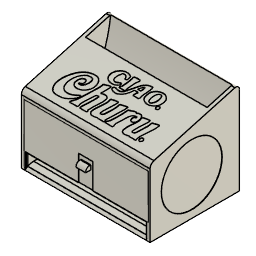
assembled chiky (Autodesk Fusion 360 design; units mm, degrees)
part number: 2026-06-02-16-31-48-869
part number: 2026-06-07-23-37-08-054
Autodesk Fusion 360 part; units mm, degrees
note: some values were not read from the file. Chosen so that the rebuilt part matches the saved one: that a step has no effect.
(part 1 of 7)
sketch "Sketch1" plane through (0, 0, 0) normal (0, 0, 1) x (1, 0, 0)
  line L0 (-170, 30) -> (0, 30)
  line L1 (0, 30) -> (0, 0)
  line L2 (0, 0) -> (-170, 0)
  line L3 (-170, 0) -> (-170, 30)
  spline S0 degree 3 poles (7.5215, 61.624) (7.5215, 61.5088) (7.5215, 61.3936) (7.5215, 61.2749) knots 0 0 0 0 1 1 1 1
  constraint horizontal L0
  constraint vertical L1
  constraint horizontal L2
  constraint vertical L3
  constraint coincident L1.end L2.start
sketch "Sketch2" plane through (0, 0, 15) normal (0, 0, 1) x (-1, 0, 0)
  line L0 (170, 0) -> (0, 0)
  line L1 (0, 0) -> (0, -30)
  line L2 (0, -30) -> (170, -30)
  line L3 (170, -30) -> (170, 0)
  line L4 (0, 0) -> (170, 0)
  line L5 (170, 0) -> (170, 30)
  line L6 (170, 30) -> (0, 30)
  line L7 (0, 30) -> (0, 0)
  constraint horizontal L4
  constraint vertical L5
  constraint horizontal L6
  constraint vertical L7
  constraint coincident L0.end L1.start
sketch "Sketch3" plane through (0, 0, 15) normal (0, 0, 1) x (-1, 0, 0)
sketch "Sketch4" plane through (0, 0, 0) normal (1, 0, 0) x (0, 1, 0)
sketch "Sketch5" plane through (0, 0, 0) normal (1, 0, 0) x (0, 1, 0)
  line L0 (0, 0) -> (-70, 0)
  line L1 (-70, 0) -> (-70, 150)
  line L2 (-70, 150) -> (0, 150)
  line L3 (0, 150) -> (0, 0)
  constraint horizontal L0
  constraint vertical L1
  constraint horizontal L2
  constraint vertical L3
  constraint coincident L0.start L3.end
sketch "Sketch6" plane through (0, 0, 0) normal (1, 0, 0) x (0, 1, 0)
sketch "Sketch7" plane through (0, 0, 0) normal (1, 0, 0) x (0, 1, 0)
sketch "Sketch8" plane through (-170, 0, 0) normal (-1, 0, 0) x (0, -1, 0)
  line L0 (0, 0) -> (70, 0)
  line L1 (70, 0) -> (70, 150)
  line L2 (70, 150) -> (0, 150)
  line L3 (0, 150) -> (0, 0)
  line L4 (0, 0) -> (70, 150)
  line L5 (0, 150) -> (0, 0)
  constraint coincident L0.start L3.end
  constraint coincident L1.end L2.start
  constraint coincident L2.end L3.start
sketch "Sketch9" plane through (0, 0, 0) normal (0, 1, 0) x (1, 0, 0)
sketch "Sketch10" plane through (0, 0, 0) normal (0, 1, 0) x (1, 0, 0)
sketch "Sketch11" plane through (0, 0, 0) normal (0, 0, 1) x (1, 0, 0)
  line L0 (100, -50) -> (-80, -50)
  line L1 (-80, -50) -> (-80, 0)
  line L2 (-80, 0) -> (100, 0)
  line L3 (100, 0) -> (100, -50)
  constraint horizontal L0
  constraint vertical L1
  constraint horizontal L2
  constraint vertical L3
sketch "Sketch12" plane through (0, 0, 0) normal (0, 0, 1) x (1, 0, 0)
  line L0 (170.2577, -0.0482) -> (0.2577, -0.0482)
  line L1 (0.2577, -0.0482) -> (0.2577, 119.9518)
  line L2 (0.2577, 119.9518) -> (170.2577, 119.9518)
  line L3 (170.2577, 119.9518) -> (170.2577, -0.0482)
  dimension "d12" = 170
  dimension "d13" = 120
  constraint horizontal L0
  constraint vertical L1
  constraint horizontal L2
  constraint vertical L3
  measures "d12" distance of L0.start L0.end
  measures "d13" distance of L0.start L2.end
sketch "Sketch13" plane through (0, 0, 0) normal (0, 1, 0) x (1, 0, 0)
sketch "Sketch14" plane through (0, 0, 0) normal (1, 0, 0) x (0, 1, 0)
sketch "Sketch15" plane through (0, 0, 0) normal (1, 0, 0) x (0, 1, 0)
sketch "Sketch16" plane through (0, 0, 0) normal (1, 0, 0) x (0, 1, 0)
  line L0 (0, 0) -> (0, 95)
  line L1 (120, 0) -> (120, 130)
  line L2 (0, 95) -> (120, 130)
  line L3 (120, 0) -> (0, 0)
  dimension "d17" = 95
  dimension "d18" = 130
  constraint coincident L0.start L3.end
  constraint vertical L0
  constraint vertical L1
  constraint perpendicular L0 L3
  measures "d17" distance of L0.start L0.end
  measures "d18" distance of L1.start L1.end
sketch "Sketch17" plane through (0, 0, 0) normal (0, 0, 1) x (1, 0, 0)
  line L0 (-15, 10) -> (160, 10)
  line L1 (160, 10) -> (160, -115)
  line L2 (160, -115) -> (-15, -115)
  line L3 (-15, -115) -> (-15, 10)
  dimension "d21" = 175
  dimension "d22" = 125
  constraint horizontal L0
  constraint vertical L1
  constraint horizontal L2
  constraint vertical L3
  measures "d21" distance of L0.start L0.end
  measures "d22" distance of L0.start L2.end
sketch "Sketch18" plane through (0, 0, 0) normal (0, 0, 1) x (1, 0, 0)
sketch "Sketch19" plane through (0, 0, 0) normal (1, 0, 0) x (0, 1, 0)
sketch "Sketch20" plane through (0, 0, 0) normal (1, 0, 0) x (0, 1, 0)
  line L0 (-115, 0) -> (-115, 125)
  line L1 (10, 0) -> (10, 90)
  line L2 (-115, 125) -> (10, 90)
  line L3 (10, 0) -> (-115, 0)
  dimension "d25" = 125
  dimension "d26" = 90
  constraint vertical L0
  constraint vertical L1
  constraint perpendicular L0 L3
  measures "d25" distance of L0.start L0.end
  measures "d26" distance of L1.start L1.end
sketch "Sketch21" plane through (0, 0, 5.436) normal (0, 0, 1) x (-1, 0, 0)
sketch "Sketch22" plane through (0, 0, 0) normal (0, 0, 1) x (1, 0, 0)
sketch "Sketch23" plane through (0, 0, 0) normal (0, 0, 1) x (1, 0, 0)
  line L0 (72.8809, -51.407) -> (-107.1191, -51.407)
  line L1 (-107.1191, -51.407) -> (-107.1191, 73.593)
  line L2 (-107.1191, 73.593) -> (72.8809, 73.593)
  line L3 (72.8809, 73.593) -> (72.8809, -51.407)
  dimension "d31" = 180
  dimension "d32" = 125
  constraint horizontal L0
  constraint vertical L1
  constraint horizontal L2
  constraint vertical L3
  measures "d31" distance of L0.start L0.end
  measures "d32" distance of L0.start L2.end
sketch "Sketch24" plane through (0, 0, 0) normal (1, 0, 0) x (0, 1, 0)
  line L0 (73.3896, -0.0085) -> (73.3896, 124.9915)
  line L1 (-51.3811, -0.081) -> (-51.3811, 89.919)
  line L2 (-51.3811, 89.919) -> (73.3896, 124.9915)
  line L3 (-51.3811, -0.081) -> (73.3896, -0.0085)
  dimension "d35" = 125
  dimension "d36" = 90
  constraint vertical L0
  constraint vertical L1
  measures "d35" distance of L0.start L0.end
  measures "d36" distance of L1.start L1.end
sketch "Sketch25" plane through (5, 0, 0) normal (1, 0, 0) x (0, 1, 0)
  line L0 (73.3896, -0.0085) -> (73.3896, 124.9915)
  line L1 (73.3896, 124.9915) -> (-51.3811, 89.919)
  line L2 (-51.3811, 89.919) -> (-51.3811, -0.081)
  line L3 (-51.3811, -0.081) -> (73.3896, -0.0085)
sketch "Sketch26" plane through (0, 0, 0) normal (1, 0, 0) x (0, 1, 0)
extrude "Extrude13" [no effect]
extrude "Extrude14" [no effect]
extrude "Extrude15" [no effect]
sketch "Sketch27" plane through (0, 0, 5) normal (0, 0, 1) x (-1, 0, 0)
sketch "Sketch28" plane through (0, 0, 0) normal (1, 0, 0) x (0, 1, 0)
  line L0 (-51.3812, -0.0812) -> (-51.3812, 89.9187)
  line L1 (-51.3812, 89.9187) -> (73.5895, 125.0479)
  line L2 (73.5895, 125.0479) -> (73.593, 0)
  line L3 (73.593, 0) -> (-51.3812, -0.0812)
  constraint vertical L0
sketch "Sketch29" plane through (0, 0, 0) normal (0, 1, 0) x (1, 0, 0)
  line L0 (-107.1194, 0) -> (73, 0)
  line L1 (73, 0) -> (73, -125)
  line L2 (73, -125) -> (-107.1194, -125)
  line L3 (-107.1194, -125) -> (-107.1194, 0)
  constraint horizontal L0
  constraint vertical L1
  constraint horizontal L2
  constraint vertical L3
sketch "Sketch30" plane through (0, 0, 5) normal (0, 0, 1) x (-1, 0, 0)
sketch "Sketch31" plane through (-107.12, 0, 0) normal (-1, 0, 0) x (0, -1, 0)
  line L0 (51.3812, -0.0812) -> (51.3812, 89.9187)
  line L1 (51.3812, 89.9187) -> (-73.5895, 125.0479)
  line L2 (-73.5895, 125.0479) -> (-73.593, 0)
  line L3 (51.3812, 89.9187) -> (51.3812, 84.9187)
  line L4 (-73.5895, 125.0479) -> (-73.5896, 120.0479)
  line L5 (-73.5896, 120.0479) -> (51.3812, 84.9187)
  line L6 (51.3812, 89.9187) -> (-73.5895, 125.0479)
  line L7 (-73.593, 0) -> (51.3812, -0.0812)
  dimension "d61" = 5
  dimension "d63" = 5
  constraint coincident L0.end L1.start
  constraint coincident L0 L3.end
  constraint coincident L1.end L2.start
  constraint parallel L2 L4
  measures "d61" distance of L0.end L3.end
  measures "d63" distance of L1.end L4.end
sketch "Sketch32" plane through (0, 0, 0) normal (1, 0, 0) x (0, 1, 0)
  line L0 (73.5937, 125.0883) -> (42.3174, 116.2538)
  line L1 (42.3174, 116.2538) -> (43.6766, 111.4421)
  line L2 (43.6766, 111.4421) -> (73.9826, 120.0025)
  line L3 (73.9826, 120.0025) -> (73.9826, 125)
  line L4 (73.9826, 125) -> (73.5937, 125.0883)
  dimension "d66" = 32.5
  dimension "d67" = 5
  constraint perpendicular L0 L1
  constraint perpendicular L1 L2
  constraint vertical L3
  measures "d66" distance of L0.start L0.end
  measures "d67" distance of L0.end L1.end
sketch "Sketch33" plane through (0, 0, 0) normal (0, 1, 0) x (1, 0, 0)
sketch "Sketch34" plane through (0, 0, 0) normal (0, 0, 1) x (1, 0, 0)
  line L0 (17.502, -9.4862) -> (-162.498, -9.4862)
  line L1 (-162.498, -9.4862) -> (-162.498, 115.5138)
  line L2 (-162.498, 115.5138) -> (17.502, 115.5138)
  line L3 (17.502, 115.5138) -> (17.502, -9.4862)
  dimension "d72" = 180
  dimension "d73" = 125
  constraint horizontal L0
  constraint vertical L1
  constraint horizontal L2
  constraint vertical L3
  measures "d72" distance of L0.start L0.end
  measures "d73" distance of L0.start L2.end
extrude "Extrude21" add sketch "Sketch34" along normal blind 130 makes body 1
shell "Shell1" thickness 5 removed faces 2 at (-102.498, 32.1805, 130) at (-102.498, 32.1805, 0) on bodies 1
sketch "Sketch35" plane through (0, 0, 0) normal (1, 0, 0) x (0, 1, 0)
sketch "Sketch36" plane through (12.502, 0, 0) normal (-1, 0, 0) x (0, -1, 0)
sketch "Sketch37" plane through (17.502, 0, 0) normal (1, 0, 0) x (0, 1, 0)
  line L0 (-9.4862, 0) -> (115.5138, 0)
  line L1 (115.5138, 0) -> (115.5138, 130)
  line L2 (115.5138, 130) -> (-9.4862, 130)
  line L3 (-9.4862, 130) -> (-9.4862, 0)
  line L4 (-9.4862, 130) -> (-9.4862, 95)
  line L5 (-9.4862, 130) -> (115.5138, 130)
  line L6 (115.5138, 130) -> (-9.4862, 130)
  line L7 (-9.4862, 95) -> (115.5138, 130)
  dimension "d79" = 35
  constraint coincident L2.end L3.start
  constraint perpendicular L2 L4
  constraint coincident L1.end L2.start
  measures "d79" distance of L2.end L4.end
extrude "Extrude22" cut sketch "Sketch37" along normal mid plane 520 contours L2 L3 L4 L5 L6 L7 bodies 1
sketch "Sketch38" plane through (0, 0, 0) normal (0, 0, 1) x (1, 0, 0)
sketch "Sketch39" plane through (0, 0, 0) normal (0, 0, -1) x (1, 0, 0)
  line L0 (12.502, 4.4862) -> (12.502, -110.5138)
  line L1 (12.502, -110.5138) -> (-157.498, -110.5138)
  line L2 (-157.498, -110.5138) -> (-157.498, 4.4862)
  line L3 (-157.498, 4.4862) -> (12.502, 4.4862)
  line L4 (-162.498, -115.5138) -> (17.502, -115.5138)
  line L5 (17.502, -115.5138) -> (17.502, 9.4862)
  line L6 (17.502, 9.4862) -> (-162.498, 9.4862)
  line L7 (-162.498, 9.4862) -> (-162.498, -115.5138)
  line L8 (17.502, 9.4862) -> (-162.498, 9.4862)
  line L9 (-162.498, 9.4862) -> (-162.498, -115.5138)
  line L10 (-162.498, -115.5138) -> (17.502, -115.5138)
  line L11 (17.502, -115.5138) -> (17.502, 9.4862)
  constraint horizontal L8
  constraint vertical L9
  constraint horizontal L10
  constraint vertical L11
  constraint coincident L4.start L7.end
  constraint coincident L5.end L6.start
sketch "Sketch40" plane through (0, 0, 0) normal (0, 0, 1) x (1, 0, 0)
sketch "Sketch41" plane through (0, 0, 0) normal (0, 0, -1) x (1, 0, 0)
extrude "Extrude23" add sketch "Sketch39" against normal blind 5 bodies 1
sketch "Sketch42" plane through (0, 0, 0) normal (0, 0, -1) x (1, 0, 0)
  line L0 (12.502, 4.4862) -> (12.502, -110.5138)
  line L1 (12.502, -110.5138) -> (-157.498, -110.5138)
  line L2 (-157.498, -110.5138) -> (-157.498, 4.4862)
  line L3 (-157.498, 4.4862) -> (12.502, 4.4862)
  line L4 (-162.498, -115.5138) -> (17.502, -115.5138)
  line L5 (17.502, -115.5138) -> (17.502, 9.4862)
  line L6 (17.502, 9.4862) -> (-162.498, 9.4862)
  line L7 (-162.498, 9.4862) -> (-162.498, -115.5138)
  line L8 (17.502, 9.4862) -> (-162.498, 9.4862)
  line L9 (17.502, -115.5138) -> (17.502, 9.4862)
  line L10 (-162.498, -115.5138) -> (17.502, -115.5138)
  line L11 (-162.498, 9.4862) -> (-162.498, -115.5138)
extrude "Extrude24" add sketch "Sketch42" against normal blind 5 contours L0 L1 L2 L3 | L4 L5 L6 L7 L8 L9 L10 L11 bodies 1
sketch "Sketch43" plane through (0, -25.3558, 90.5565) normal (0, -0.26963, 0.962964) x (1, 0, 0)
  line L0 (12.502, 141.0953) -> (12.502, 21.6723)
  line L1 (12.502, 21.6723) -> (-157.498, 21.6723)
  line L2 (-157.498, 21.6723) -> (-157.498, 141.0953)
  line L3 (-157.498, 141.0953) -> (12.502, 141.0953)
  line L4 (17.502, 16.48) -> (17.502, 146.2876)
  line L5 (17.502, 146.2876) -> (-162.498, 146.2876)
  line L6 (-162.498, 146.2876) -> (-162.498, 16.48)
  line L7 (-162.498, 16.48) -> (17.502, 16.48)
  line L8 (17.502, 146.2876) -> (17.502, 16.48)
  line L9 (17.502, 16.48) -> (-162.498, 16.48)
  line L10 (-162.498, 16.48) -> (-162.498, 146.2876)
  line L11 (17.502, 146.2876) -> (-162.498, 146.2876)
  line L12 (17.502, 104.5953) -> (-162.498, 104.5953)
  dimension "d86" = 36.5
  constraint coincident L4 L12.start
  constraint coincident L6 L12.end
  constraint perpendicular L6 L12
  measures "d86" distance of L3 L12
sketch "Sketch44" plane through (0, -25.3558, 90.5565) normal (0, -0.26963, 0.962964) x (1, 0, 0)
sketch "Sketch45" plane through (0, -25.3558, 90.5565) normal (0, -0.26963, 0.962964) x (1, 0, 0)
extrude "Extrude25" add sketch "Sketch43" against normal blind 5 contours L0 L1 L2 L4 L6 L7 L8 L9 L10 L12 | L0 L1 L2 L12 bodies 1
sketch "Sketch46" plane through (0, 0, 0) normal (0, 0, 1) x (1, 0, 0)
move_body "Move4" bodies 1 to x (1, 0, 0) y (0, 1, 0) z (0, 0, 1) at (-7.0435, -6.5956, -61.1492)
sketch "Sketch47" plane through (0, 0, 0) normal (0, 0, 1) x (1, 0, 0)
sketch "Sketch48" plane through (0, 0, 0) normal (0, 0, 1) x (1, 0, 0)
sketch "Sketch49" plane through (0, 0, 0) normal (0, 0, 1) x (1, 0, 0)
sketch "Sketch50" plane through (0, 0, 0) normal (0, 1, 0) x (1, 0, 0)
move_body "Move5" bodies 1 to x (1, 0, 0) y (0, 1, 0) z (0, 0, 1) at (0, -71.6445, -40.8297)
sketch "Sketch51" plane through (0, 0, 0) normal (0, 1, 0) x (1, 0, 0)
sketch "Sketch52" plane through (0, 37.2737, 0) normal (0, 1, 0) x (-1, 0, 0)
sketch "Sketch53" plane through (0, 37.2737, 0) normal (0, 1, 0) x (-1, 0, 0)
sketch "Sketch54" plane through (0, 0, 0) normal (0, 1, 0) x (1, 0, 0)
sketch "Sketch55" plane through (0, 0, 0) normal (1, 0, 0) x (0, 1, 0)
sketch "Sketch56" plane through (0, 0, 0) normal (1, 0, 0) x (0, 1, 0)
move_body "Move6" bodies 1 to x (1, 0, 0) y (0, 1, 0) z (0, 0, 1) at (0, 0, 50)
sketch "Sketch57" plane through (0, 0, 0) normal (0, 0, 1) x (1, 0, 0)
move_body "Move7" bodies 1 to x (1, 0, 0) y (0, 1, 0) z (0, 0, 1) at (80, 0, 0)
sketch "Sketch58" plane through (0, 0, 0) normal (1, 0, 0) x (0, 1, 0)
sketch "Sketch61" plane through (-89.5415, 0, 0) normal (-1, 0, 0) x (0, -1, 0)
  line L0 (87.7263, 43.0211) -> (-37.2737, 78.0211)
  line L1 (-37.2737, 78.0211) -> (-37.2737, -51.9789)
  line L2 (-37.2737, -51.9789) -> (87.7263, -51.9789)
  line L3 (87.7263, -51.9789) -> (87.7263, 43.0211)
  line L4 (-37.2737, -51.9789) -> (-37.2737, 78.0211)
  line L5 (87.7263, -51.9789) -> (-37.2737, -51.9789)
  line L6 (87.7263, -51.9789) -> (87.7263, 43.0211)
  line L7 (-37.2737, -51.9789) -> (-37.2737, 4.0211)
  line L8 (-37.2737, -51.9789) -> (47.7263, -51.9789)
  line L9 (-37.2737, 4.0211) -> (47.7263, -51.9789)
  line L10 (-37.2737, 4.0211) -> (-37.2737, -51.9789)
  line L11 (47.7263, -51.9789) -> (-37.2737, -51.9789)
  dimension "d92" = 56
  dimension "d93" = 85
  constraint coincident L1.end L2.start
  constraint perpendicular L2 L7
  constraint coincident L2 L8.end
  measures "d92" distance of L1.end L7.end
  measures "d93" distance of L1.end L8.end
sketch "Sketch62" plane through (-89.5415, 0, 0) normal (-1, 0, 0) x (0, -1, 0)
extrude "Extrude26" add sketch "Sketch61" against normal blind 180 contours L1 L2 L4 L5 L7 L8 L9 L10 L11 bodies 1
sketch "Sketch63" plane through (0, 37.2737, 0) normal (0, 1, 0) x (-1, 0, 0)
move_body "Move8" bodies 1 to x (1, 0, 0) y (0, 1, 0) z (0, 0, 1) at (0, 48.1482, 13.4815)
sketch "Sketch64" plane through (0, -39.5781, 0) normal (0, -1, 0) x (1, 0, 0)
move_body "Move9" bodies 1 to x (1, 0, 0) y (0, 1, 0) z (0, 0, 1) at (0, -28.8889, -8.0889)
sketch "Sketch65" plane through (0, -68.467, 0) normal (0, -1, 0) x (1, 0, 0)
move_body "Move10" bodies 1 to x (1, 0, 0) y (0, 1, 0) z (0, 0, 1) at (0, -38.5186, -10.7852)
sketch "Sketch66" plane through (0, 0, 0) normal (0, 1, 0) x (1, 0, 0)
sketch "Sketch67" plane through (0, -106.9856, 0) normal (0, -1, 0) x (1, 0, 0)
sketch "Sketch68" plane through (0, -106.9856, 0) normal (0, -1, 0) x (1, 0, 0)
move_body "Move11" bodies 1 to x (1, 0, 0) y (0, 1, 0) z (0, 0, 1) at (0, 0, 180)
move_body "Move12" bodies 1 to x (1, 0, 0) y (0, 1, 0) z (0, 0, 1) at (-9.5745, 43.535, 39.5174)
move_body "Move13" bodies 1 to x (1, 0, 0) y (0, 1, 0) z (0, 0, 1) at (-4.2434, 5.0858, -145.3116)
sketch "Sketch69" plane through (0, -58.3648, 0) normal (0, -1, 0) x (1, 0, 0)
  line L0 (76.6406, 111.8343) -> (-103.3594, 111.8343)
  line L1 (-103.3594, 16.8343) -> (76.6406, 16.8343)
sketch "Sketch70" plane through (0, 0, 0) normal (0, 1, 0) x (1, 0, 0)
sketch "Sketch71" plane through (0, -58.3648, 0) normal (0, -1, 0) x (1, 0, 0)
sketch "Sketch72" plane through (0, 61.6352, 0) normal (0, -1, 0) x (1, 0, 0)
  line L0 (-98.3594, 69.5402) -> (71.6406, 69.5402)
  line L1 (71.6406, 69.5402) -> (71.6406, 145.4343)
  line L2 (71.6406, 145.4343) -> (-98.3594, 145.4343)
  line L3 (-98.3594, 145.4343) -> (-98.3594, 69.5402)
sketch "Sketch73" plane through (0, -58.3648, 0) normal (0, -1, 0) x (1, 0, 0)
  line L0 (76.6406, 16.8343) -> (76.6406, 111.8343)
sketch "Sketch74" plane through (0, 0, 0) normal (0, 1, 0) x (1, 0, 0)
sketch "Sketch75" plane through (0, 0, 0) normal (0, 1, 0) x (1, 0, 0)
sketch "Sketch76" plane through (0, -58.3648, 0) normal (0, -1, 0) x (1, 0, 0)
  line L0 (-103.3594, 16.8343) -> (76.6406, 16.8343)
sketch "Sketch77" plane through (0, -58.3648, 0) normal (0, -1, 0) x (1, 0, 0)
  line L0 (71.6406, 21.8343) -> (-98.3594, 21.8343)
  line L1 (-98.3594, 21.8343) -> (-98.3594, 39.3343)
  line L2 (-98.3594, 39.3343) -> (71.6406, 39.3343)
  line L3 (71.6406, 39.3343) -> (71.6406, 21.8343)
  line L4 (76.6406, 16.8343) -> (76.6406, 111.8343)
  line L5 (-103.3594, 16.8343) -> (76.6406, 16.8343)
  dimension "d106" = 170
  dimension "d107" = 17.5
  dimension "d108" = 5
  dimension "d109" = 5
  constraint horizontal L0
  constraint vertical L1
  constraint horizontal L2
  constraint vertical L3
  measures "d106" distance of L0.start L0.end
  measures "d107" distance of L0.start L2.end
  measures "d108" distance of L3 L4
  measures "d109" distance of L0 L5
extrude "Extrude27" cut sketch "Sketch77" against normal blind 20 bodies 1
fillet "Fillet2" radius 17.5 1 edges at (-13.3594, -58.3648, 21.8343) on bodies 1
sketch "Sketch78" plane through (0, -58.3648, 0) normal (0, -1, 0) x (1, 0, 0)
  line L0 (76.6406, 111.8343) -> (-103.3594, 111.8343)
  line L1 (76.6406, 16.8343) -> (76.6406, 111.8343)
  line L2 (-103.3594, 111.8343) -> (-103.3594, 16.8343)
sketch "Sketch79" plane through (0, -58.3648, 0) normal (0, -1, 0) x (1, 0, 0)
sketch "Sketch80" plane through (0, -58.3648, 0) normal (0, -1, 0) x (1, 0, 0)
sketch "Sketch81" plane through (0, -58.3648, 0) normal (0, -1, 0) x (1, 0, 0)
  line L0 (-103.3594, 111.8343) -> (-103.3594, 16.8343)
  line L1 (76.6406, 111.8343) -> (-103.3594, 111.8343)
  line L2 (76.6406, 16.8343) -> (76.6406, 111.8343)
  line L3 (-98.3594, 39.3343) -> (71.6406, 39.3343)
  line L4 (-3.3594, 39.3343) -> (-23.3594, 39.3343)
  line L5 (-23.3594, 39.3343) -> (-23.3594, 86.8343)
  line L6 (-23.3594, 86.8343) -> (-3.3594, 86.8343)
  line L7 (-3.3594, 86.8343) -> (-3.3594, 39.3343)
  arc A0 (-3.3594, 86.8343) -> (-23.3594, 86.8343) centre (-13.3594, 86.8343) ccw
  dimension "d121" = 20
  dimension "d122" = 47.5
  dimension "d123" = 80
  constraint horizontal L4
  constraint vertical L5
  constraint horizontal L6
  constraint vertical L7
  constraint coincident L3 L4.start
  constraint tangent L7 A0
  measures "d121" distance of L4.start L4.end
  measures "d122" distance of L4.start L6.end
  measures "d123" distance of L0 L5
extrude "Extrude28" cut sketch "Sketch81" against normal blind 5 bodies 1
fillet "Fillet3" radius 175 1 edges at (-13.3594, 61.6352, 69.5402) on bodies 1
sketch "Sketch82" plane through (0, -58.3648, 0) normal (0, -1, 0) x (1, 0, 0)
sketch "Sketch83" plane through (0, -33.2802, 118.858) normal (0, -0.26963, 0.962964) x (1, 0, 0)
  line L0 (-98.3594, 62.066) -> (-98.3594, 98.566)
  line L1 (-98.3594, 98.566) -> (71.6406, 98.566)
  line L2 (71.6406, 98.566) -> (71.6406, 62.066)
  line L3 (71.6406, 62.066) -> (-98.3594, 62.066)
  line L4 (-103.3594, 103.7583) -> (-103.3594, -26.0493)
  line L5 (-103.3594, -26.0493) -> (76.6406, -26.0493)
  line L6 (76.6406, -26.0493) -> (76.6406, 103.7583)
  line L7 (76.6406, 103.7583) -> (-103.3594, 103.7583)
  spline S0 degree 3 poles (-46.4635, 26.2376) (-45.3943, 25.3067) (-45.3943, 25.3067) (-44.5627, 24.3057) knots 0 0 0 0 1 1 1 1
  spline S1 degree 3 poles (-44.5627, 24.3057) (-44.1414, 23.8141) (-44.1414, 23.8141) (-43.7117, 23.3125) knots 0 0 0 0 1 1 1 1
  spline S2 degree 3 poles (-43.7117, 23.3125) (-41.7397, 20.4716) (-41.5438, 17.6346) (-41.9764, 14.2723) knots 0 0 0 0 1 1 1 1
  spline S3 degree 3 poles (-41.9764, 14.2723) (-43.3271, 10.0635) (-45.7689, 7.5657) (-49.5171, 5.3917) knots 0 0 0 0 1 1 1 1
  spline S4 degree 3 poles (-49.5171, 5.3917) (-52.778, 4.0448) (-56.1727, 3.7927) (-59.5505, 4.862) knots 0 0 0 0 1 1 1 1
  spline S5 degree 3 poles (-59.5505, 4.862) (-61.5726, 5.7138) (-62.4831, 6.7703) (-63.4144, 8.7881) knots 0 0 0 0 1 1 1 1
  spline S6 degree 3 poles (-63.4144, 8.7881) (-63.851, 11.7357) (-63.0022, 13.8359) (-61.4201, 16.2665) knots 0 0 0 0 1 1 1 1
  spline S7 degree 3 poles (-61.4201, 16.2665) (-60.1525, 17.6652) (-59.5525, 17.7466) (-57.6498, 17.9803) knots 0 0 0 0 1 1 1 1
  spline S8 degree 3 poles (-57.6498, 17.9803) (-55.936, 17.7622) (-55.936, 17.7622) (-54.9389, 16.9208) knots 0 0 0 0 1 1 1 1
  spline S9 degree 3 poles (-54.9389, 16.9208) (-54.2933, 15.428) (-54.3698, 14.7928) (-54.9389, 13.2751) knots 0 0 0 0 1 1 1 1
  spline S10 degree 3 poles (-54.9389, 13.2751) (-56.0005, 11.9102) (-56.6269, 11.3644) (-58.3042, 10.907) knots 0 0 0 0 1 1 1 1
  spline S11 degree 3 poles (-58.3042, 10.907) (-58.6743, 10.8659) (-59.0445, 10.8247) (-59.4259, 10.7824) knots 0 0 0 0 1 1 1 1
  spline S12 degree 3 poles (-59.4259, 10.7824) (-59.2614, 10.4533) (-59.0969, 10.1243) (-58.9274, 9.7853) knots 0 0 0 0 1 1 1 1
  spline S13 degree 3 poles (-58.9274, 9.7853) (-57.0546, 9.6069) (-56.066, 9.7177) (-54.378, 10.5954) knots 0 0 0 0 1 1 1 1
  spline S14 degree 3 poles (-54.378, 10.5954) (-51.916, 12.6293) (-50.6703, 14.7313) (-50.3331, 17.8712) knots 0 0 0 0 1 1 1 1
  spline S15 degree 3 poles (-50.3331, 17.8712) (-50.2741, 19.6846) (-50.2681, 20.9096) (-51.1374, 22.5296) knots 0 0 0 0 1 1 1 1
  spline S16 degree 3 poles (-51.1374, 22.5296) (-53.5345, 23.8423) (-56.0472, 23.6463) (-58.6313, 22.8996) knots 0 0 0 0 1 1 1 1
  spline S17 degree 3 poles (-58.6313, 22.8996) (-63.3775, 20.9654) (-66.17, 17.8363) (-68.3999, 13.2751) knots 0 0 0 0 1 1 1 1
  spline S18 degree 3 poles (-68.3999, 13.2751) (-70.2091, 8.9562) (-70.6779, 4.5741) (-69.0543, 0.1257) knots 0 0 0 0 1 1 1 1
  spline S19 degree 3 poles (-69.0543, 0.1257) (-67.9163, -2.3898) (-66.6272, -4.0487) (-64.131, -5.3272) knots 0 0 0 0 1 1 1 1
  spline S20 degree 3 poles (-64.131, -5.3272) (-56.9412, -6.7652) (-51.5834, -4.234) (-45.4663, -0.6844) knots 0 0 0 0 1 1 1 1
  spline S21 degree 3 poles (-45.4663, -0.6844) (-44.9094, -2.5384) (-44.9094, -2.5384) (-45.4352, -3.8004) knots 0 0 0 0 1 1 1 1
  spline S22 degree 3 poles (-45.4352, -3.8004) (-49.1382, -8.7377) (-53.8993, -12.1669) (-59.9245, -13.6469) knots 0 0 0 0 1 1 1 1
  spline S23 degree 3 poles (-59.9245, -13.6469) (-61.6648, -13.8653) (-63.3753, -13.9076) (-65.1281, -13.8962) knots 0 0 0 0 1 1 1 1
  spline S24 degree 3 poles (-65.1281, -13.8962) (-65.5868, -13.8958) (-66.0455, -13.8955) (-66.518, -13.8952) knots 0 0 0 0 1 1 1 1
  spline S25 degree 3 poles (-66.518, -13.8952) (-69.9194, -13.8203) (-72.6076, -13.2463) (-75.3797, -11.1541) knots 0 0 0 0 1 1 1 1
  spline S26 degree 3 poles (-75.3797, -11.1541) (-75.3797, -10.825) (-75.3797, -10.496) (-75.3797, -10.157) knots 0 0 0 0 1 1 1 1
  spline S27 degree 3 poles (-75.3797, -10.157) (-75.8733, -9.9925) (-76.3668, -9.8279) (-76.8754, -9.6584) knots 0 0 0 0 1 1 1 1
  spline S28 degree 3 poles (-76.8754, -9.6584) (-79.7359, -5.1153) (-79.688, -0.5102) (-78.7625, 4.6692) knots 0 0 0 0 1 1 1 1
  spline S29 degree 3 poles (-78.7625, 4.6692) (-76.8721, 12.5224) (-72.0494, 19.991) (-65.2664, 24.4381) knots 0 0 0 0 1 1 1 1
  spline S30 degree 3 poles (-65.2664, 24.4381) (-59.4161, 27.9062) (-52.8229, 29.5775) (-46.4635, 26.2376) knots 0 0 0 0 1 1 1 1
  spline S31 degree 3 poles (-27.5183, 25.2405) (-28.2733, 21.0185) (-29.3748, 16.9083) (-30.5097, 12.7766) knots 0 0 0 0 1 1 1 1
  spline S32 degree 3 poles (-30.5097, 12.7766) (-30.1498, 12.9379) (-29.7899, 13.0992) (-29.4191, 13.2654) knots 0 0 0 0 1 1 1 1
  spline S33 degree 3 poles (-29.4191, 13.2654) (-26.7908, 14.2182) (-24.058, 14.2347) (-21.5045, 13.0882) knots 0 0 0 0 1 1 1 1
  spline S34 degree 3 poles (-21.5045, 13.0882) (-20.5385, 12.278) (-20.5385, 12.278) (-20.04, 11.2809) knots 0 0 0 0 1 1 1 1
  spline S35 degree 3 poles (-20.04, 11.2809) (-19.8884, 8.4584) (-20.1929, 6.3486) (-21.113, 3.6448) knots 0 0 0 0 1 1 1 1
  spline S36 degree 3 poles (-21.113, 3.6448) (-21.2225, 3.3157) (-21.332, 2.9866) (-21.4448, 2.6475) knots 0 0 0 0 1 1 1 1
  spline S37 degree 3 poles (-21.4448, 2.6475) (-21.7915, 1.6076) (-22.1459, 0.5706) (-22.5016, -0.4663) knots 0 0 0 0 1 1 1 1
  spline S38 degree 3 poles (-22.5016, -0.4663) (-22.8544, -1.5053) (-23.2054, -2.5447) (-23.5531, -3.5854) knots 0 0 0 0 1 1 1 1
  spline S39 degree 3 poles (-23.5531, -3.5854) (-23.8686, -4.5286) (-24.1898, -5.4699) (-24.5113, -6.4111) knots 0 0 0 0 1 1 1 1
  spline S40 degree 3 poles (-24.5113, -6.4111) (-25.0321, -8.1852) (-25.3097, -9.8215) (-25.5241, -11.6527) knots 0 0 0 0 1 1 1 1
  spline S41 degree 3 poles (-25.5241, -11.6527) (-25.0305, -11.8172) (-24.537, -11.9817) (-24.0284, -12.1512) knots 0 0 0 0 1 1 1 1
  spline S42 degree 3 poles (-24.0284, -12.1512) (-24.2752, -12.8916) (-24.2752, -12.8916) (-24.527, -13.6469) knots 0 0 0 0 1 1 1 1
  spline S43 degree 3 poles (-24.527, -13.6469) (-27.8175, -13.6469) (-31.1079, -13.6469) (-34.4981, -13.6469) knots 0 0 0 0 1 1 1 1
  spline S44 degree 3 poles (-34.4981, -13.6469) (-35.0613, -11.3941) (-34.8788, -11.0226) (-33.9995, -8.9729) knots 0 0 0 0 1 1 1 1
  spline S45 degree 3 poles (-33.9995, -8.9729) (-32.7356, -5.8434) (-31.6406, -2.6809) (-30.6031, 0.5308) knots 0 0 0 0 1 1 1 1
  spline S46 degree 3 poles (-30.6031, 0.5308) (-30.4466, 1.0031) (-30.2902, 1.4754) (-30.1289, 1.962) knots 0 0 0 0 1 1 1 1
  spline S47 degree 3 poles (-30.1289, 1.962) (-29.3801, 4.3001) (-28.8021, 6.2998) (-29.014, 8.7881) knots 0 0 0 0 1 1 1 1
  spline S48 degree 3 poles (-29.014, 8.7881) (-30.4802, 8.6963) (-30.4802, 8.6963) (-32.0053, 8.2896) knots 0 0 0 0 1 1 1 1
  spline S49 degree 3 poles (-32.0053, 8.2896) (-33.5782, 5.8311) (-34.2952, 2.7561) (-35.2351, 0.0012) knots 0 0 0 0 1 1 1 1
  spline S50 degree 3 poles (-35.2351, 0.0012) (-35.4697, -0.6812) (-35.7081, -1.3624) (-35.9503, -2.0422) knots 0 0 0 0 1 1 1 1
  spline S51 degree 3 poles (-35.9503, -2.0422) (-37.3268, -5.9085) (-38.3302, -9.0424) (-37.4894, -13.1483) knots 0 0 0 0 1 1 1 1
  spline S52 degree 3 poles (-37.4894, -13.1483) (-37.988, -13.6469) (-37.988, -13.6469) (-39.0514, -13.7035) knots 0 0 0 0 1 1 1 1
  spline S53 degree 3 poles (-39.0514, -13.7035) (-39.5083, -13.7009) (-39.9652, -13.6983) (-40.436, -13.6956) knots 0 0 0 0 1 1 1 1
  spline S54 degree 3 poles (-40.436, -13.6956) (-40.9292, -13.694) (-41.4225, -13.6923) (-41.9307, -13.6907) knots 0 0 0 0 1 1 1 1
  spline S55 degree 3 poles (-41.9307, -13.6907) (-42.4496, -13.6865) (-42.9686, -13.6823) (-43.5033, -13.678) knots 0 0 0 0 1 1 1 1
  spline S56 degree 3 poles (-43.5033, -13.678) (-44.0242, -13.6758) (-44.545, -13.6735) (-45.0817, -13.6712) knots 0 0 0 0 1 1 1 1
  spline S57 degree 3 poles (-45.0817, -13.6712) (-46.3732, -13.6653) (-47.6647, -13.6571) (-48.9562, -13.6469) knots 0 0 0 0 1 1 1 1
  spline S58 degree 3 poles (-48.9562, -13.6469) (-48.9562, -11.5033) (-48.9553, -11.4675) (-47.6475, -10.0323) knots 0 0 0 0 1 1 1 1
  spline S59 degree 3 poles (-47.6475, -10.0323) (-43.7177, -4.9602) (-42.3223, 2.2188) (-40.3561, 8.2584) knots 0 0 0 0 1 1 1 1
  spline S60 degree 3 poles (-40.3561, 8.2584) (-40.1912, 8.7635) (-40.1912, 8.7635) (-40.0229, 9.2788) knots 0 0 0 0 1 1 1 1
  spline S61 degree 3 poles (-40.0229, 9.2788) (-37.6437, 16.1116) (-37.6437, 16.1116) (-36.9909, 23.2463) knots 0 0 0 0 1 1 1 1
  spline S62 degree 3 poles (-36.9909, 23.2463) (-35.6941, 23.6775) (-34.3959, 24.1024) (-33.0959, 24.5238) knots 0 0 0 0 1 1 1 1
  spline S63 degree 3 poles (-33.0959, 24.5238) (-32.728, 24.6469) (-32.3601, 24.77) (-31.981, 24.8968) knots 0 0 0 0 1 1 1 1
  spline S64 degree 3 poles (-31.981, 24.8968) (-29.1834, 25.7955) (-29.1834, 25.7955) (-27.5183, 25.2405) knots 0 0 0 0 1 1 1 1
  spline S65 degree 3 poles (6.3835, 14.7708) (6.1127, 12.0428) (5.6003, 9.5956) (4.6892, 7.0042) knots 0 0 0 0 1 1 1 1
  spline S66 degree 3 poles (4.6892, 7.0042) (4.5717, 6.6589) (4.4542, 6.3136) (4.3332, 5.9577) knots 0 0 0 0 1 1 1 1
  spline S67 degree 3 poles (4.3332, 5.9577) (3.9608, 4.8642) (3.5835, 3.7724) (3.2052, 2.6808) knots 0 0 0 0 1 1 1 1
  spline S68 degree 3 poles (3.2052, 2.6808) (1.5696, -2.0596) (0.0086, -6.7523) (-1.0949, -11.6527) knots 0 0 0 0 1 1 1 1
  spline S69 degree 3 poles (-1.0949, -11.6527) (-0.7658, -11.6527) (-0.4368, -11.6527) (-0.0977, -11.6527) knots 0 0 0 0 1 1 1 1
  spline S70 degree 3 poles (-0.0977, -11.6527) (-0.2623, -12.3107) (-0.4268, -12.9688) (-0.5963, -13.6469) knots 0 0 0 0 1 1 1 1
  spline S71 degree 3 poles (-0.5963, -13.6469) (-1.9881, -13.6603) (-3.3798, -13.6702) (-4.7717, -13.678) knots 0 0 0 0 1 1 1 1
  spline S72 degree 3 poles (-4.7717, -13.678) (-5.1676, -13.6822) (-5.5635, -13.6864) (-5.9714, -13.6907) knots 0 0 0 0 1 1 1 1
  spline S73 degree 3 poles (-5.9714, -13.6907) (-8.9588, -13.7034) (-8.9588, -13.7034) (-10.0689, -13.1483) knots 0 0 0 0 1 1 1 1
  spline S74 degree 3 poles (-10.0689, -13.1483) (-10.9001, -13.3977) (-11.7313, -13.6475) (-12.5616, -13.9) knots 0 0 0 0 1 1 1 1
  spline S75 degree 3 poles (-12.5616, -13.9) (-14.7875, -14.4478) (-16.8229, -14.4674) (-18.9494, -13.5222) knots 0 0 0 0 1 1 1 1
  spline S76 degree 3 poles (-18.9494, -13.5222) (-20.8709, -11.985) (-20.8709, -11.985) (-21.5356, -10.6555) knots 0 0 0 0 1 1 1 1
  spline S77 degree 3 poles (-21.5356, -10.6555) (-21.3134, -8.1621) (-20.7022, -5.9589) (-19.8803, -3.6018) knots 0 0 0 0 1 1 1 1
  spline S78 degree 3 poles (-19.8803, -3.6018) (-19.6521, -2.9293) (-19.4242, -2.2568) (-19.1967, -1.5842) knots 0 0 0 0 1 1 1 1
  spline S79 degree 3 poles (-19.1967, -1.5842) (-18.8406, -0.5415) (-18.4818, 0.5001) (-18.1166, 1.5396) knots 0 0 0 0 1 1 1 1
  spline S80 degree 3 poles (-18.1166, 1.5396) (-16.1856, 7.0289) (-16.1856, 7.0289) (-16.5501, 12.7766) knots 0 0 0 0 1 1 1 1
  spline S81 degree 3 poles (-16.5501, 12.7766) (-9.7531, 14.4937) (-9.7531, 14.4937) (-6.579, 14.2723) knots 0 0 0 0 1 1 1 1
  spline S82 degree 3 poles (-6.579, 14.2723) (-6.8843, 9.8661) (-8.4956, 5.9019) (-9.9501, 1.7636) knots 0 0 0 0 1 1 1 1
  spline S83 degree 3 poles (-9.9501, 1.7636) (-10.9837, -1.2371) (-11.8432, -3.993) (-12.0631, -7.1656) knots 0 0 0 0 1 1 1 1
  spline S84 degree 3 poles (-12.0631, -7.1656) (-10.5924, -7.8391) (-10.5924, -7.8391) (-9.3041, -7.1286) knots 0 0 0 0 1 1 1 1
  spline S85 degree 3 poles (-9.3041, -7.1286) (-7.7904, -5.9466) (-7.4573, -5.081) (-6.8497, -3.2707) knots 0 0 0 0 1 1 1 1
  spline S86 degree 3 poles (-6.8497, -3.2707) (-6.6553, -2.6929) (-6.4609, -2.1152) (-6.2606, -1.5199) knots 0 0 0 0 1 1 1 1
  spline S87 degree 3 poles (-6.2606, -1.5199) (-5.9709, -0.6128) (-5.9709, -0.6128) (-5.6753, 0.3127) knots 0 0 0 0 1 1 1 1
  spline S88 degree 3 poles (-5.6753, 0.3127) (-5.3712, 1.1967) (-5.3712, 1.1967) (-5.0609, 2.0985) knots 0 0 0 0 1 1 1 1
  spline S89 degree 3 poles (-5.0609, 2.0985) (-3.8631, 5.7504) (-3.2922, 8.9359) (-3.5876, 12.7766) knots 0 0 0 0 1 1 1 1
  spline S90 degree 3 poles (-3.5876, 12.7766) (-3.1011, 12.8788) (-2.6146, 12.981) (-2.1134, 13.0862) knots 0 0 0 0 1 1 1 1
  spline S91 degree 3 poles (-2.1134, 13.0862) (-1.4791, 13.2206) (-0.8448, 13.3549) (-0.1912, 13.4933) knots 0 0 0 0 1 1 1 1
  spline S92 degree 3 poles (-0.1912, 13.4933) (0.7545, 13.6928) (0.7545, 13.6928) (1.7193, 13.8964) knots 0 0 0 0 1 1 1 1
  spline S93 degree 3 poles (1.7193, 13.8964) (5.6111, 14.7708) (5.6111, 14.7708) (6.3835, 14.7708) knots 0 0 0 0 1 1 1 1
  spline S94 degree 3 poles (51.2535, 14.7708) (50.968, 11.8083) (50.3452, 9.1752) (49.4151, 6.3538) knots 0 0 0 0 1 1 1 1
  spline S95 degree 3 poles (49.4151, 6.3538) (49.2842, 5.946) (49.1533, 5.5383) (49.0184, 5.1181) knots 0 0 0 0 1 1 1 1
  spline S96 degree 3 poles (49.0184, 5.1181) (48.6035, 3.8268) (48.1839, 2.5371) (47.7636, 1.2475) knots 0 0 0 0 1 1 1 1
  spline S97 degree 3 poles (47.7636, 1.2475) (47.3438, -0.0458) (46.9251, -1.3394) (46.5088, -2.6338) knots 0 0 0 0 1 1 1 1
  spline S98 degree 3 poles (46.5088, -2.6338) (46.2508, -3.4358) (45.9907, -4.2371) (45.7281, -5.0377) knots 0 0 0 0 1 1 1 1
  spline S99 degree 3 poles (45.7281, -5.0377) (44.78, -7.9768) (43.9588, -10.5737) (44.7723, -13.6469) knots 0 0 0 0 1 1 1 1
  spline S100 degree 3 poles (44.7723, -13.6469) (43.2974, -13.6603) (41.8226, -13.6702) (40.3476, -13.678) knots 0 0 0 0 1 1 1 1
  spline S101 degree 3 poles (40.3476, -13.678) (39.9279, -13.6822) (39.5083, -13.6864) (39.0759, -13.6907) knots 0 0 0 0 1 1 1 1
  spline S102 degree 3 poles (39.0759, -13.6907) (38.6742, -13.6923) (38.2726, -13.6939) (37.8587, -13.6956) knots 0 0 0 0 1 1 1 1
  spline S103 degree 3 poles (37.8587, -13.6956) (37.3026, -13.6995) (37.3026, -13.6995) (36.7353, -13.7035) knots 0 0 0 0 1 1 1 1
  spline S104 degree 3 poles (36.7353, -13.7035) (35.7983, -13.6469) (35.7983, -13.6469) (34.8012, -13.1483) knots 0 0 0 0 1 1 1 1
  spline S105 degree 3 poles (34.8012, -13.1483) (34.2768, -13.3026) (33.7523, -13.4568) (33.212, -13.6157) knots 0 0 0 0 1 1 1 1
  spline S106 degree 3 poles (33.212, -13.6157) (30.5857, -14.3476) (28.7126, -14.5154) (26.1699, -13.4599) knots 0 0 0 0 1 1 1 1
  spline S107 degree 3 poles (26.1699, -13.4599) (24.8301, -12.6498) (24.8301, -12.6498) (23.8329, -11.6527) knots 0 0 0 0 1 1 1 1
  spline S108 degree 3 poles (23.8329, -11.6527) (23.2791, -7.0262) (25.1473, -2.9513) (26.7261, 1.3088) knots 0 0 0 0 1 1 1 1
  spline S109 degree 3 poles (26.7261, 1.3088) (28.1258, 5.1163) (29.2424, 8.2139) (28.32, 12.278) knots 0 0 0 0 1 1 1 1
  spline S110 degree 3 poles (28.32, 12.278) (31.4838, 13.7069) (34.818, 14.4504) (38.2911, 14.2723) knots 0 0 0 0 1 1 1 1
  spline S111 degree 3 poles (38.2911, 14.2723) (38.0188, 11.558) (37.5256, 9.1961) (36.6357, 6.6011) knots 0 0 0 0 1 1 1 1
  spline S112 degree 3 poles (36.6357, 6.6011) (36.4077, 5.9212) (36.1799, 5.2412) (35.9521, 4.5611) knots 0 0 0 0 1 1 1 1
  spline S113 degree 3 poles (35.9521, 4.5611) (35.5942, 3.5069) (35.2342, 2.4535) (34.872, 1.4007) knots 0 0 0 0 1 1 1 1
  spline S114 degree 3 poles (34.872, 1.4007) (34.52, 0.373) (34.1753, -0.6569) (33.8313, -1.6874) knots 0 0 0 0 1 1 1 1
  spline S115 degree 3 poles (33.8313, -1.6874) (33.623, -2.2964) (33.4147, -2.9055) (33.2001, -3.533) knots 0 0 0 0 1 1 1 1
  spline S116 degree 3 poles (33.2001, -3.533) (32.8072, -5.1704) (32.8209, -6.073) (33.3055, -7.6642) knots 0 0 0 0 1 1 1 1
  spline S117 degree 3 poles (33.3055, -7.6642) (35.1778, -7.4112) (36.1068, -7.1508) (37.294, -5.67) knots 0 0 0 0 1 1 1 1
  spline S118 degree 3 poles (37.294, -5.67) (38.1053, -3.76) (38.7197, -1.7882) (39.3512, 0.1879) knots 0 0 0 0 1 1 1 1
  spline S119 degree 3 poles (39.3512, 0.1879) (39.6593, 1.1452) (39.9805, 2.0973) (40.3028, 3.0499) knots 0 0 0 0 1 1 1 1
  spline S120 degree 3 poles (40.3028, 3.0499) (41.371, 6.3535) (42.1231, 8.868) (41.2824, 12.278) knots 0 0 0 0 1 1 1 1
  spline S121 degree 3 poles (41.2824, 12.278) (48.3772, 14.7708) (48.3772, 14.7708) (51.2535, 14.7708) knots 0 0 0 0 1 1 1 1
  spline S122 degree 3 poles (18.3488, 14.7708) (18.5956, 14.0305) (18.5956, 14.0305) (18.8474, 13.2751) knots 0 0 0 0 1 1 1 1
  spline S123 degree 3 poles (18.8474, 13.2751) (19.1764, 13.5219) (19.5055, 13.7687) (19.8445, 14.023) knots 0 0 0 0 1 1 1 1
  spline S124 degree 3 poles (19.8445, 14.023) (21.7354, 14.9684) (23.2516, 15.2282) (25.3286, 14.7708) knots 0 0 0 0 1 1 1 1
  spline S125 degree 3 poles (25.3286, 14.7708) (26.9337, 13.5072) (27.674, 12.7203) (28.32, 10.7824) knots 0 0 0 0 1 1 1 1
  spline S126 degree 3 poles (28.32, 10.7824) (28.4814, 7.8759) (28.2625, 5.9661) (26.4192, 3.6779) knots 0 0 0 0 1 1 1 1
  spline S127 degree 3 poles (26.4192, 3.6779) (25.1645, 2.6742) (24.4352, 2.3869) (22.8358, 2.3069) knots 0 0 0 0 1 1 1 1
  spline S128 degree 3 poles (22.8358, 2.3069) (21.7141, 2.5562) (21.7141, 2.5562) (20.8416, 3.304) knots 0 0 0 0 1 1 1 1
  spline S129 degree 3 poles (20.8416, 3.304) (20.3431, 4.9867) (20.3431, 4.9867) (20.3431, 6.7939) knots 0 0 0 0 1 1 1 1
  spline S130 degree 3 poles (20.3431, 6.7939) (21.2467, 8.0091) (21.2467, 8.0091) (22.3373, 8.7881) knots 0 0 0 0 1 1 1 1
  spline S131 degree 3 poles (22.3373, 8.7881) (22.6663, 8.7881) (22.9954, 8.7881) (23.3344, 8.7881) knots 0 0 0 0 1 1 1 1
  spline S132 degree 3 poles (23.3344, 8.7881) (23.3344, 9.2817) (23.3344, 9.7753) (23.3344, 10.2838) knots 0 0 0 0 1 1 1 1
  spline S133 degree 3 poles (23.3344, 10.2838) (20.7001, 10.0772) (19.1909, 9.7296) (17.3517, 7.791) knots 0 0 0 0 1 1 1 1
  spline S134 degree 3 poles (17.3517, 7.791) (15.4573, 4.4284) (14.3353, 0.9081) (13.2075, -2.7721) knots 0 0 0 0 1 1 1 1
  spline S135 degree 3 poles (13.2075, -2.7721) (13.0221, -3.3515) (12.8367, -3.9309) (12.6456, -4.5278) knots 0 0 0 0 1 1 1 1
  spline S136 degree 3 poles (12.6456, -4.5278) (12.4731, -5.0866) (12.3005, -5.6454) (12.1227, -6.2211) knots 0 0 0 0 1 1 1 1
  spline S137 degree 3 poles (12.1227, -6.2211) (11.9657, -6.7257) (11.8087, -7.2304) (11.6469, -7.7503) knots 0 0 0 0 1 1 1 1
  spline S138 degree 3 poles (11.6469, -7.7503) (11.3486, -9.2638) (11.498, -10.172) (11.8676, -11.6527) knots 0 0 0 0 1 1 1 1
  spline S139 degree 3 poles (11.8676, -11.6527) (11.8676, -12.3107) (11.8676, -12.9688) (11.8676, -13.6469) knots 0 0 0 0 1 1 1 1
  spline S140 degree 3 poles (11.8676, -13.6469) (8.2481, -13.6469) (4.6286, -13.6469) (0.8994, -13.6469) knots 0 0 0 0 1 1 1 1
  spline S141 degree 3 poles (0.8994, -13.6469) (0.8994, -12.9888) (0.8994, -12.3307) (0.8994, -11.6527) knots 0 0 0 0 1 1 1 1
  spline S142 degree 3 poles (0.8994, -11.6527) (1.2835, -11.271) (1.6677, -10.8893) (2.0635, -10.4961) knots 0 0 0 0 1 1 1 1
  spline S143 degree 3 poles (2.0635, -10.4961) (3.5988, -8.952) (4.0463, -7.7897) (4.7086, -5.7284) knots 0 0 0 0 1 1 1 1
  spline S144 degree 3 poles (4.7086, -5.7284) (4.8146, -5.4019) (4.9205, -5.0754) (5.0297, -4.739) knots 0 0 0 0 1 1 1 1
  spline S145 degree 3 poles (5.0297, -4.739) (5.2511, -4.0505) (5.4688, -3.3607) (5.6829, -2.6699) knots 0 0 0 0 1 1 1 1
  spline S146 degree 3 poles (5.6829, -2.6699) (6.0064, -1.6294) (6.3438, -0.5942) (6.6834, 0.4412) knots 0 0 0 0 1 1 1 1
  spline S147 degree 3 poles (6.6834, 0.4412) (7.8898, 4.1988) (8.7651, 7.8084) (8.8763, 11.7795) knots 0 0 0 0 1 1 1 1
  spline S148 degree 3 poles (8.8763, 11.7795) (9.3393, 11.9288) (9.3393, 11.9288) (9.8117, 12.0811) knots 0 0 0 0 1 1 1 1
  spline S149 degree 3 poles (9.8117, 12.0811) (11.679, 12.6854) (13.5042, 13.3111) (15.2952, 14.1165) knots 0 0 0 0 1 1 1 1
  spline S150 degree 3 poles (15.2952, 14.1165) (16.8532, 14.7708) (16.8532, 14.7708) (18.3488, 14.7708) knots 0 0 0 0 1 1 1 1
  spline S151 degree 3 poles (6.4458, 48.7038) (6.8995, 48.6993) (7.3533, 48.6948) (7.8207, 48.6902) knots 0 0 0 0 1 1 1 1
  spline S152 degree 3 poles (7.8207, 48.6902) (8.3432, 48.6815) (8.3432, 48.6815) (8.8763, 48.6726) knots 0 0 0 0 1 1 1 1
  spline S153 degree 3 poles (8.8763, 48.6726) (9.6809, 45.2226) (8.9834, 42.0856) (8.3777, 38.6392) knots 0 0 0 0 1 1 1 1
  spline S154 degree 3 poles (8.3777, 38.6392) (8.1763, 37.4857) (7.9788, 36.3315) (7.7857, 35.1766) knots 0 0 0 0 1 1 1 1
  spline S155 degree 3 poles (7.7857, 35.1766) (7.6963, 34.6688) (7.607, 34.161) (7.515, 33.6378) knots 0 0 0 0 1 1 1 1
  spline S156 degree 3 poles (7.515, 33.6378) (7.379, 32.2034) (7.5684, 31.1227) (7.8792, 29.7275) knots 0 0 0 0 1 1 1 1
  spline S157 degree 3 poles (7.8792, 29.7275) (7.3806, 29.2289) (7.3806, 29.2289) (5.587, 29.1803) knots 0 0 0 0 1 1 1 1
  spline S158 degree 3 poles (5.587, 29.1803) (4.845, 29.1836) (4.103, 29.1895) (3.361, 29.1978) knots 0 0 0 0 1 1 1 1
  spline S159 degree 3 poles (3.361, 29.1978) (2.7937, 29.2012) (2.7937, 29.2012) (2.2149, 29.2046) knots 0 0 0 0 1 1 1 1
  spline S160 degree 3 poles (2.2149, 29.2046) (1.2778, 29.2105) (0.3408, 29.2194) (-0.5963, 29.2289) knots 0 0 0 0 1 1 1 1
  spline S161 degree 3 poles (-0.5963, 29.2289) (-0.5963, 31.6192) (0.0177, 33.0074) (0.8994, 35.2116) knots 0 0 0 0 1 1 1 1
  spline S162 degree 3 poles (0.8994, 35.2116) (-0.9104, 35.2116) (-2.7201, 35.2116) (-4.5847, 35.2116) knots 0 0 0 0 1 1 1 1
  spline S163 degree 3 poles (-4.5847, 35.2116) (-4.7698, 34.5638) (-4.9549, 33.916) (-5.1456, 33.2485) knots 0 0 0 0 1 1 1 1
  spline S164 degree 3 poles (-5.1456, 33.2485) (-6.7823, 28.3843) (-9.766, 24.8591) (-14.1819, 22.3115) knots 0 0 0 0 1 1 1 1
  spline S165 degree 3 poles (-14.1819, 22.3115) (-17.5313, 21.3067) (-20.6928, 21.1634) (-23.8726, 22.7477) knots 0 0 0 0 1 1 1 1
  spline S166 degree 3 poles (-23.8726, 22.7477) (-24.4176, 23.0768) (-24.9626, 23.4058) (-25.5241, 23.7448) knots 0 0 0 0 1 1 1 1
  spline S167 degree 3 poles (-25.5241, 23.7448) (-25.5454, 24.5755) (-25.5444, 25.4069) (-25.5241, 26.2376) knots 0 0 0 0 1 1 1 1
  spline S168 degree 3 poles (-25.5241, 26.2376) (-25.0255, 26.7362) (-25.0255, 26.7362) (-23.8103, 26.8296) knots 0 0 0 0 1 1 1 1
  spline S169 degree 3 poles (-23.8103, 26.8296) (-22.274, 26.7488) (-21.0525, 26.5096) (-19.5726, 26.1441) knots 0 0 0 0 1 1 1 1
  spline S170 degree 3 poles (-19.5726, 26.1441) (-17.1011, 25.6328) (-15.7463, 25.8465) (-13.5588, 27.2347) knots 0 0 0 0 1 1 1 1
  spline S171 degree 3 poles (-13.5588, 27.2347) (-11.0348, 29.6653) (-9.4534, 32.5656) (-7.8565, 35.6478) knots 0 0 0 0 1 1 1 1
  spline S172 degree 3 poles (-7.8565, 35.6478) (-3.2892, 44.4606) (-3.2892, 44.4606) (0.8059, 46.9277) knots 0 0 0 0 1 1 1 1
  spline S173 degree 3 poles (0.8059, 46.9277) (1.366, 47.2747) (1.366, 47.2747) (1.9374, 47.6288) knots 0 0 0 0 1 1 1 1
  spline S174 degree 3 poles (1.9374, 47.6288) (3.5884, 48.5703) (4.538, 48.7282) (6.4458, 48.7038) knots 0 0 0 0 1 1 1 1
  spline S175 degree 3 poles (1.8965, 44.1856) (1.2149, 43.4849) (0.5534, 42.7646) (-0.0977, 42.0356) knots 0 0 0 0 1 1 1 1
  spline S176 degree 3 poles (-0.0977, 42.0356) (-0.4576, 41.6365) (-0.8175, 41.2374) (-1.1883, 40.8262) knots 0 0 0 0 1 1 1 1
  spline S177 degree 3 poles (-1.1883, 40.8262) (-2.1801, 39.722) (-2.1801, 39.722) (-2.5905, 38.2029) knots 0 0 0 0 1 1 1 1
  spline S178 degree 3 poles (-2.5905, 38.2029) (-0.595, 38.1572) (-0.595, 38.1572) (1.3979, 38.2029) knots 0 0 0 0 1 1 1 1
  spline S179 degree 3 poles (1.3979, 38.2029) (2.2652, 39.0702) (2.0819, 40.2937) (2.1769, 41.4747) knots 0 0 0 0 1 1 1 1
  spline S180 degree 3 poles (2.1769, 41.4747) (2.2187, 41.9792) (2.2605, 42.4837) (2.3035, 43.0035) knots 0 0 0 0 1 1 1 1
  spline S181 degree 3 poles (2.3035, 43.0035) (2.3337, 43.3936) (2.3639, 43.7837) (2.395, 44.1856) knots 0 0 0 0 1 1 1 1
  spline S182 degree 3 poles (2.395, 44.1856) (2.2305, 44.1856) (2.066, 44.1856) (1.8965, 44.1856) knots 0 0 0 0 1 1 1 1
  spline S183 degree 3 poles (28.1018, 47.8313) (30.2357, 46.551) (31.4142, 45.0334) (32.4642, 42.7834) knots 0 0 0 0 1 1 1 1
  spline S184 degree 3 poles (32.4642, 42.7834) (33.145, 39.6269) (32.4793, 36.9391) (30.9549, 34.158) knots 0 0 0 0 1 1 1 1
  spline S185 degree 3 poles (30.9549, 34.158) (28.831, 31.04) (25.9739, 29.5097) (22.3373, 28.7304) knots 0 0 0 0 1 1 1 1
  spline S186 degree 3 poles (22.3373, 28.7304) (18.8675, 28.3586) (15.8092, 29.3013) (12.8959, 31.1608) knots 0 0 0 0 1 1 1 1
  spline S187 degree 3 poles (12.8959, 31.1608) (11.0255, 33.0879) (10.7248, 35.0485) (10.7147, 37.6732) knots 0 0 0 0 1 1 1 1
  spline S188 degree 3 poles (10.7147, 37.6732) (10.7894, 40.7322) (11.1826, 42.483) (13.3769, 44.7153) knots 0 0 0 0 1 1 1 1
  spline S189 degree 3 poles (13.3769, 44.7153) (17.5169, 48.5729) (22.5945, 50.3883) (28.1018, 47.8313) knots 0 0 0 0 1 1 1 1
  spline S190 degree 3 poles (18.8474, 43.1885) (17.3812, 40.5494) (16.9836, 37.162) (17.7568, 34.2457) knots 0 0 0 0 1 1 1 1
  spline S191 degree 3 poles (17.7568, 34.2457) (18.2408, 32.6927) (18.2408, 32.6927) (19.3459, 31.7217) knots 0 0 0 0 1 1 1 1
  spline S192 degree 3 poles (19.3459, 31.7217) (21.3952, 31.7217) (22.1815, 32.0787) (23.7083, 33.4667) knots 0 0 0 0 1 1 1 1
  spline S193 degree 3 poles (23.7083, 33.4667) (25.8751, 36.3954) (25.9968, 39.7145) (25.5701, 43.2158) knots 0 0 0 0 1 1 1 1
  spline S194 degree 3 poles (25.5701, 43.2158) (25.3486, 44.3377) (25.3486, 44.3377) (24.3315, 45.6813) knots 0 0 0 0 1 1 1 1
  spline S195 degree 3 poles (24.3315, 45.6813) (21.5872, 46.1692) (20.5347, 45.2976) (18.8474, 43.1885) knots 0 0 0 0 1 1 1 1
  spline S196 degree 3 poles (-21.3097, 47.1146) (-21.0552, 46.9707) (-20.8007, 46.8267) (-20.5385, 46.6784) knots 0 0 0 0 1 1 1 1
  spline S197 degree 3 poles (-20.5385, 46.6784) (-20.5116, 45.8684) (-20.4923, 45.0582) (-20.4762, 44.2479) knots 0 0 0 0 1 1 1 1
  spline S198 degree 3 poles (-20.4762, 44.2479) (-20.4647, 43.7968) (-20.4531, 43.3456) (-20.4412, 42.8808) knots 0 0 0 0 1 1 1 1
  spline S199 degree 3 poles (-20.4412, 42.8808) (-20.5385, 41.6928) (-20.5385, 41.6928) (-21.5356, 40.6957) knots 0 0 0 0 1 1 1 1
  spline S200 degree 3 poles (-21.5356, 40.6957) (-22.5016, 40.6646) (-22.5016, 40.6646) (-23.5299, 41.1943) knots 0 0 0 0 1 1 1 1
  spline S201 degree 3 poles (-23.5299, 41.1943) (-24.0628, 42.3422) (-24.5628, 43.5062) (-25.0255, 44.6842) knots 0 0 0 0 1 1 1 1
  spline S202 degree 3 poles (-25.0255, 44.6842) (-26.2248, 45.2838) (-26.9948, 45.2329) (-28.3285, 45.2139) knots 0 0 0 0 1 1 1 1
  spline S203 degree 3 poles (-28.3285, 45.2139) (-28.7359, 45.2094) (-29.1434, 45.2049) (-29.5632, 45.2003) knots 0 0 0 0 1 1 1 1
  spline S204 degree 3 poles (-29.5632, 45.2003) (-29.8755, 45.1945) (-30.1879, 45.1887) (-30.5097, 45.1827) knots 0 0 0 0 1 1 1 1
  spline S205 degree 3 poles (-30.5097, 45.1827) (-32.0959, 42.0724) (-33.4072, 39.2858) (-33.0024, 35.7102) knots 0 0 0 0 1 1 1 1
  spline S206 degree 3 poles (-33.0024, 35.7102) (-32.1313, 33.8515) (-32.1313, 33.8515) (-30.5097, 32.7188) knots 0 0 0 0 1 1 1 1
  spline S207 degree 3 poles (-30.5097, 32.7188) (-28.5314, 32.4888) (-27.3912, 32.703) (-25.7422, 33.7471) knots 0 0 0 0 1 1 1 1
  spline S208 degree 3 poles (-25.7422, 33.7471) (-24.0284, 34.7131) (-24.0284, 34.7131) (-22.5639, 34.5884) knots 0 0 0 0 1 1 1 1
  spline S209 degree 3 poles (-22.5639, 34.5884) (-22.2246, 34.465) (-21.8853, 34.3416) (-21.5356, 34.2145) knots 0 0 0 0 1 1 1 1
  spline S210 degree 3 poles (-21.5356, 34.2145) (-21.5668, 33.0927) (-21.5668, 33.0927) (-22.0342, 31.7217) knots 0 0 0 0 1 1 1 1
  spline S211 degree 3 poles (-22.0342, 31.7217) (-23.224, 30.9052) (-24.2316, 30.3133) (-25.5241, 29.7275) knots 0 0 0 0 1 1 1 1
  spline S212 degree 3 poles (-25.5241, 29.7275) (-25.9765, 29.5116) (-26.429, 29.2956) (-26.8951, 29.0731) knots 0 0 0 0 1 1 1 1
  spline S213 degree 3 poles (-26.8951, 29.0731) (-29.8903, 28.4396) (-32.8233, 28.7933) (-35.6822, 29.8521) knots 0 0 0 0 1 1 1 1
  spline S214 degree 3 poles (-35.6822, 29.8521) (-37.8313, 31.2849) (-39.4754, 32.8138) (-40.4808, 35.2116) knots 0 0 0 0 1 1 1 1
  spline S215 degree 3 poles (-40.4808, 35.2116) (-40.9233, 37.9489) (-40.5428, 40.3215) (-39.1818, 42.7308) knots 0 0 0 0 1 1 1 1
  spline S216 degree 3 poles (-39.1818, 42.7308) (-34.8163, 48.735) (-27.9216, 50.4909) (-21.3097, 47.1146) knots 0 0 0 0 1 1 1 1
  spline S217 degree 3 poles (-12.7486, 48.7038) (-12.2203, 48.7004) (-12.2203, 48.7004) (-11.6814, 48.697) knots 0 0 0 0 1 1 1 1
  spline S218 degree 3 poles (-11.6814, 48.697) (-10.8115, 48.6911) (-9.9416, 48.6821) (-9.0717, 48.6726) knots 0 0 0 0 1 1 1 1
  spline S219 degree 3 poles (-9.0717, 48.6726) (-8.729, 47.8313) (-8.729, 47.8313) (-8.5732, 46.6784) knots 0 0 0 0 1 1 1 1
  spline S220 degree 3 poles (-8.5732, 46.6784) (-8.8044, 46.3005) (-9.0356, 45.9226) (-9.2738, 45.5333) knots 0 0 0 0 1 1 1 1
  spline S221 degree 3 poles (-9.2738, 45.5333) (-10.1164, 44.105) (-10.397, 43.039) (-10.6687, 41.4124) knots 0 0 0 0 1 1 1 1
  spline S222 degree 3 poles (-10.6687, 41.4124) (-10.7998, 40.6316) (-10.7998, 40.6316) (-10.9335, 39.8349) knots 0 0 0 0 1 1 1 1
  spline S223 degree 3 poles (-10.9335, 39.8349) (-11.0184, 39.2964) (-11.1032, 38.7578) (-11.1906, 38.2029) knots 0 0 0 0 1 1 1 1
  spline S224 degree 3 poles (-11.1906, 38.2029) (-11.2832, 37.6644) (-11.3757, 37.1258) (-11.4711, 36.571) knots 0 0 0 0 1 1 1 1
  spline S225 degree 3 poles (-11.4711, 36.571) (-11.876, 34.0861) (-12.0998, 32.2002) (-11.5645, 29.7275) knots 0 0 0 0 1 1 1 1
  spline S226 degree 3 poles (-11.5645, 29.7275) (-12.0631, 29.2289) (-12.0631, 29.2289) (-13.8567, 29.1803) knots 0 0 0 0 1 1 1 1